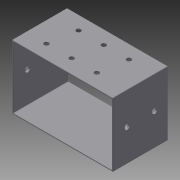
# Autodesk Inventor part: Box Base
Saved by Autodesk Inventor 2014 (Build 180170000, 170)
## iProperties
Created: 2014-05-19
Part Number: Box Base
Material: Generic
Document SubType Name: Modeling
Designer: lpluta-ehlers
Density: 1 g/cm^3
Appearance: Default
Author: lpluta-ehlers
Autodesk Inventor part; units mm, degrees
ref_plane "YZ Plane" through (0, 0, 0) normal (1, 0, 0) x (0, 1, 0)
ref_plane "XZ Plane" through (0, 0, 0) normal (0, 1, 0) x (-1, 0, 0)
ref_plane "XY Plane" through (0, 0, 0) normal (0, 0, 1) x (1, 0, 0)
sketch "Sketch1" plane through (0, 0, 0) normal (0, 1, 0) x (-1, 0, 0)
  line L0 (0, 0) -> (-279.4, 0)
  line L1 (-279.4, 0) -> (-279.4, -152.4)
  line L2 (-279.4, -152.4) -> (0, -152.4)
  line L3 (0, -152.4) -> (0, 0)
  dimension "blength" = 279.4
  dimension "bwidth" = 152.4
  constraints: 8 end point, 2 parallel, 1 horizontal, 1 perpendicular
  measures "blength" distance of L1.end L2.end
  measures "bwidth" distance of L0.end L1.end
extrude "Extrusion1" add sketch "Sketch1" along normal blind 177.8
shell "Shell1" thickness 3.81 removed faces 2 at (93.1333, 118.5333, 0) at (186.2667, 118.5333, -152.4)
sketch "Sketch2" plane through (279.4, 0, 0) normal (1, 0, 0) x (0, 0, -1)
  line L0 (0, 0) -> (152.4, 0) projected
  line L1 (152.4, 0) -> (152.4, 177.8) projected
  line L2 (0, 177.8) -> (152.4, 177.8) projected
  line L3 (0, 0) -> (0, 177.8) projected
  circle A0 centre (38.1, 88.9) radius 6.35
  circle A1 centre (114.3, 88.9) radius 6.35
  line L4 (76.2, 177.8) -> (76.2, 0) construction
  line L5 (38.1, 177.8) -> (38.1, 50.8) construction
  line L6 (114.3, 177.8) -> (114.3, 50.8) construction
  line L7 (0, 88.9) -> (152.4, 88.9) construction
  dimension "csize" = 12.7
  dimension "d6" = 12.7
  dimension "sidecirclemasterxloc" = 76.2
  dimension "sidecirclexloc" = 38.1
  dimension "sidecircle2xloc" = 38.1
  dimension "sidecircleyloc" = 88.9
  dimension "d11" = 0
  dimension "d12" = 127
  dimension "d13" = 0
  dimension "d14" = 127
  constraints: 8 end point, 4 midpoint, 4 point on line, 2 centre point, 2 parallel, 2 perpendicular
  measures "csize" diameter of A0
  measures "d6" diameter of A1
  measures "sidecirclemasterxloc" distance between parallel lines of L1 L4
  measures "sidecirclexloc" distance between parallel lines of L5 L4
  measures "sidecircle2xloc" distance between parallel lines of L6 L4
  measures "sidecircleyloc" distance between parallel lines of L2 L7
  measures "d11" distance from line of L6.start L2
  measures "d12" distance from line of L6.end L2
  measures "d13" distance from line of L5.start L2
  measures "d14" distance from line of L5.end L2
extrude "Extrusion2" cut sketch "Sketch2" against normal blind 304.8 contours A0 | A1
sketch "Sketch3" plane through (0, 177.8, 0) normal (0, 1, 0) x (1, 0, 0)
  line L0 (0, 152.4) -> (0, 0) projected
  line L1 (22.225, 38.1) -> (212.725, 38.1) construction
  line L2 (22.225, 114.3) -> (212.725, 114.3) construction
  line L3 (139.7, 152.4) -> (139.7, 0) construction
  line L4 (69.85, 150.6432) -> (69.85, -1.7568) construction
  line L5 (209.55, 152.4) -> (209.55, 0) construction
  circle A0 centre (69.85, 114.3) radius 6.35
  circle A1 centre (139.7, 114.3) radius 6.35
  circle A2 centre (209.55, 114.3) radius 6.35
  line L6 (196.85, 152.4) -> (196.85, 0) construction
  line L7 (127, 152.4) -> (127, 0) construction
  line L8 (57.15, 150.6432) -> (57.15, -1.7568) construction
  circle A3 centre (57.15, 38.1) radius 6.35
  circle A4 centre (127, 38.1) radius 6.35
  circle A5 centre (196.85, 38.1) radius 6.35
  dimension "TopCircDistFrmCntr" = 76.2
  dimension "topCircsDistFrmSide" = 139.7
  dimension "OtherTopCircDistFrmCntr" = 69.85
  dimension "OtherCentDist" = 139.7
  dimension "d22" = 12.7
  dimension "d23" = 12.7
  dimension "d24" = 12.7
  dimension "IndylTopDist" = 12.7
  dimension "d26" = 12.7
  dimension "d27" = 12.7
  dimension "d28" = 12.7
  dimension "d29" = 12.7
  dimension "d30" = 12.7
  constraints: 16 end point, 12 point on line, 7 parallel, 6 centre point
  measures "TopCircDistFrmCntr" distance between parallel lines of L1 L2
  measures "topCircsDistFrmSide" distance between parallel lines of L0 L3
  measures "OtherTopCircDistFrmCntr" distance between parallel lines of L4 L3
  measures "OtherCentDist" distance between parallel lines of L5 L4
  measures "d22" diameter of A0
  measures "d23" diameter of A1
  measures "d24" diameter of A2
  measures "IndylTopDist" distance between parallel lines of L5 L6
  measures "d26" distance between parallel lines of L7 L3
  measures "d27" distance between parallel lines of L8 L4
  measures "d28" diameter of A3
  measures "d29" diameter of A4
  measures "d30" diameter of A5
extrude "Extrusion3" cut sketch "Sketch3" against normal blind 50.8
sketch "Sketch7" plane through (279.4, 0, 0) normal (1, 0, 0) x (0, 0, -1)
  circle A0 centre (38.1, 88.9) radius 6.35 projected
  circle A1 centre (114.3, 88.9) radius 6.35 projected
  circle A2 centre (38.1, 88.9) radius 6.477
  circle A3 centre (114.3, 88.9) radius 6.477
  dimension "cholder" = 12.954
  dimension "d39" = 12.954
  constraints: 2 centre point, 2 coincident
  measures "cholder" diameter of A2
  measures "d39" diameter of A3
extrude "Extrusion4" add sketch "Sketch7" along normal blind 1.27 and the other way blind 5.08
sketch "Sketch8" plane through (0, 0, -152.4) normal (-1, 0, 0) x (0, 0, 1)
  circle A0 centre (114.3, 88.9) radius 6.35 projected
  circle A1 centre (38.1, 88.9) radius 6.35 projected
  circle A2 centre (38.1, 88.9) radius 6.477
  circle A3 centre (114.3, 88.9) radius 6.477
  dimension "d44" = 12.954
  dimension "d45" = 12.954
  constraints: 2 centre point, 2 coincident
  measures "d44" diameter of A2
  measures "d45" diameter of A3
extrude "Extrusion5" add sketch "Sketch8" along normal blind 1.27 and the other way blind 5.08
fillet "Fillet1" radius 1.27 24 edges at (0, 177.8, -76.2) (139.7, 177.8, -152.4) (279.4, 177.8, -76.2) (139.7, 177.8, 0) (0, 88.9, -152.4) (3.81, 88.9, -152.4) (139.7, 173.99, -152.4) (275.59, 88.9, -152.4) (279.4, 88.9, -152.4) (139.7, 3.81, -152.4) (139.7, 0, -152.4) (275.59, 3.81, -76.2) (3.81, 88.9, 0) (0, 88.9, 0) (0, 0, -76.2) (3.81, 3.81, -76.2) (275.59, 88.9, 0) (139.7, 173.99, 0) (139.7, 3.81, 0) (139.7, 0, 0) (279.4, 88.9, 0) (279.4, 0, -76.2) (3.81, 173.99, -76.2) (275.59, 173.99, -76.2)
fillet "Fillet2" radius 0.254 20 edges at (190.5, 177.8, -38.1) (120.65, 177.8, -38.1) (50.8, 177.8, -38.1) (63.5, 177.8, -114.3) (133.35, 177.8, -114.3) (203.2, 177.8, -114.3) (190.5, 173.99, -38.1) (120.65, 173.99, -38.1) (63.5, 173.99, -114.3) (133.35, 173.99, -114.3) (203.2, 173.99, -114.3) (50.8, 173.99, -38.1) (280.67, 88.9, -31.75) (280.67, 88.9, -107.95) (-1.27, 88.9, -44.45) (-1.27, 88.9, -120.65) (274.32, 88.9, -31.75) (5.08, 88.9, -44.45) (5.08, 88.9, -120.65) (274.32, 88.9, -107.95)
equation "\"d6\" = csize"
equation "\"sidecircle2xloc\" = sidecirclexloc"
equation "\"sidecircleyloc\" = 0.5 * bheight"
equation "\"topCircsDistFrmSide\" = 0.5 * blength"
equation "\"OtherTopCircDistFrmCntr\" = 0.5 * topCircsDistFrmSide"
equation "\"OtherCentDist\" = topCircsDistFrmSide"
equation "\"d22\" = csize"
equation "\"d23\" = csize"
equation "\"d24\" = csize"
equation "\"d26\" = IndylTopDist"
equation "\"d27\" = IndylTopDist"
equation "\"d28\" = csize"
equation "\"d29\" = csize"
equation "\"d30\" = csize"
equation "\"d39\" = cholder"
equation "\"d44\" = cholder"
equation "\"d45\" = cholder"
equation "\"d46\" = sideExtrusionOUT"
equation "\"d47\" = sideExtrusionIN"
equation "\"bheight\" = 177.8"
equation "\"sideExtrusionOUT\" = 1.27"
equation "\"sideExtrusionIN\" = 5.08"
body "Solid1"
